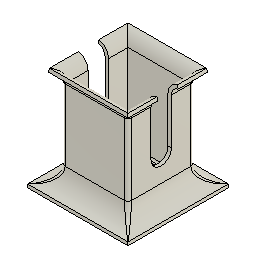
Butter Stick v2 (Autodesk Fusion 360 design; units mm, degrees)
Autodesk Fusion 360 part; units mm, degrees
sketch "Sketch1" plane through (0, 0, 0) normal (0, 0, 1) x (1, 0, 0)
  line L0 (17.5, -17.5) -> (-17.5, -17.5)
  line L1 (-17.5, -17.5) -> (-17.5, 17.5)
  line L2 (-17.5, 17.5) -> (17.5, 17.5)
  line L3 (17.5, 17.5) -> (17.5, -17.5)
  line L4 (17.5, -17.5) -> (-17.5, 17.5) construction
  line L5 (-17.5, -17.5) -> (17.5, 17.5) construction
  dimension "d1" = 35
  dimension "d2" = 35
  constraint perpendicular L0 L1
  constraint parallel L0 L2
  constraint parallel L1 L3
  constraint horizontal L0
  constraint coincident L4 origin
  constraint coincident L5 origin
  measures "d1" distance of L1.end L2.end
  measures "d2" distance of L0.end L1.end
extrude "Extrude1" add sketch "Sketch1" along normal blind 50
shell "Shell1" thickness 2 outward yes removed faces 1 at (5.8333, -5.8333, 50)
sketch "Sketch2" plane through (0, 0, -2) normal (0, 0, -1) x (1, 0, 0)
  line L0 (-19.5, -19.5) -> (19.5, -19.5)
  line L1 (19.5, -19.5) -> (19.5, 19.5)
  line L2 (19.5, 19.5) -> (-19.5, 19.5)
  line L3 (-19.5, 19.5) -> (-19.5, -19.5)
  line L4 (29.5, -29.5) -> (-29.5, -29.5)
  line L5 (-29.5, -29.5) -> (-29.5, 29.5)
  line L6 (-29.5, 29.5) -> (29.5, 29.5)
  line L7 (29.5, 29.5) -> (29.5, -29.5)
  line L8 (29.5, -29.5) -> (-29.5, 29.5) construction
  line L9 (-29.5, -29.5) -> (29.5, 29.5) construction
  dimension "d6" = 10
  constraint perpendicular L4 L5
  constraint parallel L4 L6
  constraint parallel L5 L7
  constraint horizontal L4
  constraint coincident L8 origin
  constraint coincident L9 origin
  measures "d6" distance of L1 L7
extrude "Extrude2" add sketch "Sketch2" along normal blind 2 contours L0 L1 L2 L3 | L4 L5 L6 L7
fillet "Fillet1" radius 10 4 edges at (19.5, 0, -2) (0, 19.5, -2) (-19.5, 0, -2) (0, -19.5, -2)
sketch "Sketch3" plane through (0, 0, 0) normal (1, 0, 0) x (0, 1, 0)
  line L0 (17.5, 0) -> (-17.5, 0)
  line L1 (-17.5, 0) -> (-17.5, 50)
  line L2 (-17.5, 50) -> (17.5, 50)
  line L3 (17.5, 50) -> (17.5, 0)
  line L4 (19.5, 8) -> (19.5, 50)
  line L5 (19.5, 50) -> (19.5, 8)
  arc A0 (23.5, 55) -> (19.5, 50) centre (24.625, 50) ccw
  arc A1 (23.061, 56.9512) -> (17.5, 50) centre (24.625, 50) ccw
  line L6 (24.625, 50) -> (23.061, 56.9512)
  line L7 (19.5, 50) -> (17.5, 50)
  dimension "d16" = 4
  dimension "d17" = 5
  constraint tangent L5 A0
  constraint coincident L4.end L5.start
  constraint tangent L3 A1
  constraint coincident L2.end L3.start
  constraint coincident A0.centre A1.centre
  constraint coincident A0.start L6
  measures "d16" distance of L5 A0.start
  measures "d17" vertical distance of A0.start L4.end
sweep "Sweep1" add profiles "Sketch3" along 4 edges at (-17.5, 0, 50) (0, 17.5, 50) (17.5, 0, 50) (0, -17.5, 50) section 1 contours A0 A1 L6 L7
sketch "Sketch4" plane through (-19.5, 0, 0) normal (-1, 0, 0) x (0, -1, 0)
  line L0 (-19.5, 8) -> (19.5, 8)
  line L1 (19.5, 8) -> (19.5, 50)
  line L2 (19.5, 50) -> (-19.5, 50)
  line L3 (-19.5, 50) -> (-19.5, 8)
  circle A0 centre (-0.0025, 23) radius 6
  line L4 (-6.0025, 23) -> (-6.0025, 56.9512)
  line L5 (5.9975, 23) -> (5.9975, 56.9512)
  line L6 (5.9975, 56.9512) -> (-6.0025, 56.9512)
  line L7 (23.061, 56.9512) -> (-23.061, 56.9512)
  dimension "d18" = 12
  dimension "d19" = 15
  constraint coincident A0 L4.start
  constraint tangent A0 L4
  constraint coincident A0 L5.start
  constraint vertical L5
  constraint tangent A0 L5
  constraint parallel L4 L5
  constraint perpendicular L4 L6
  constraint collinear L6 L7
  measures "d18" diameter of A0
  measures "d19" distance of L0 A0.centre
extrude "Extrude3" cut sketch "Sketch4" along normal through all and the other way through all contours L2 L4 L5 L6 L7 | L2 A0 L4 L5 | A0
sketch "Sketch5" plane through (0, 0, 0) normal (0, 0, 1) x (-1, 0, 0)
  line L0 (-17.5, -17.5) -> (17.5, -17.5)
  line L1 (17.5, -17.5) -> (17.5, 17.5)
  line L2 (17.5, 17.5) -> (-17.5, 17.5)
  line L3 (-17.5, 17.5) -> (-17.5, -17.5)
  line L4 (-2, 2) -> (2, 2)
  line L5 (2, 2) -> (2, -2)
  line L6 (2, -2) -> (-2, -2)
  line L7 (-2, -2) -> (-2, 2)
  line L8 (-2, 2) -> (2, -2) construction
  line L9 (2, 2) -> (-2, -2) construction
  line L10 (-10.5, -14.5) -> (-14.5, -14.5)
  line L11 (-14.5, -14.5) -> (-14.5, -10.5)
  line L12 (-14.5, -10.5) -> (-10.5, -10.5)
  line L13 (-10.5, -10.5) -> (-10.5, -14.5)
  line L14 (-4.25, -14.5) -> (-8.25, -14.5)
  line L15 (-8.25, -14.5) -> (-8.25, -10.5)
  line L16 (-8.25, -10.5) -> (-4.25, -10.5)
  line L17 (-4.25, -10.5) -> (-4.25, -14.5)
  line L18 (2, -14.5) -> (-2, -14.5)
  line L19 (-2, -14.5) -> (-2, -10.5)
  line L20 (-2, -10.5) -> (2, -10.5)
  line L21 (2, -10.5) -> (2, -14.5)
  line L22 (8.25, -14.5) -> (4.25, -14.5)
  line L23 (4.25, -14.5) -> (4.25, -10.5)
  line L24 (4.25, -10.5) -> (8.25, -10.5)
  line L25 (8.25, -10.5) -> (8.25, -14.5)
  line L26 (14.5, -14.5) -> (10.5, -14.5)
  line L27 (10.5, -14.5) -> (10.5, -10.5)
  line L28 (10.5, -10.5) -> (14.5, -10.5)
  line L29 (14.5, -10.5) -> (14.5, -14.5)
  line L30 (-10.5, -8.25) -> (-14.5, -8.25)
  line L31 (-14.5, -8.25) -> (-14.5, -4.25)
  line L32 (-14.5, -4.25) -> (-10.5, -4.25)
  line L33 (-10.5, -4.25) -> (-10.5, -8.25)
  line L34 (-4.25, -8.25) -> (-8.25, -8.25)
  line L35 (-8.25, -8.25) -> (-8.25, -4.25)
  line L36 (-8.25, -4.25) -> (-4.25, -4.25)
  line L37 (-4.25, -4.25) -> (-4.25, -8.25)
  line L38 (2, -8.25) -> (-2, -8.25)
  line L39 (-2, -8.25) -> (-2, -4.25)
  line L40 (-2, -4.25) -> (2, -4.25)
  line L41 (2, -4.25) -> (2, -8.25)
  line L42 (8.25, -8.25) -> (4.25, -8.25)
  line L43 (4.25, -8.25) -> (4.25, -4.25)
  line L44 (4.25, -4.25) -> (8.25, -4.25)
  line L45 (8.25, -4.25) -> (8.25, -8.25)
  line L46 (14.5, -8.25) -> (10.5, -8.25)
  line L47 (10.5, -8.25) -> (10.5, -4.25)
  line L48 (10.5, -4.25) -> (14.5, -4.25)
  line L49 (14.5, -4.25) -> (14.5, -8.25)
  line L50 (-10.5, -2) -> (-14.5, -2)
  line L51 (-14.5, -2) -> (-14.5, 2)
  line L52 (-14.5, 2) -> (-10.5, 2)
  line L53 (-10.5, 2) -> (-10.5, -2)
  line L54 (-4.25, -2) -> (-8.25, -2)
  line L55 (-8.25, -2) -> (-8.25, 2)
  line L56 (-8.25, 2) -> (-4.25, 2)
  line L57 (-4.25, 2) -> (-4.25, -2)
  line L58 (8.25, -2) -> (4.25, -2)
  line L59 (4.25, -2) -> (4.25, 2)
  line L60 (4.25, 2) -> (8.25, 2)
  line L61 (8.25, 2) -> (8.25, -2)
  line L62 (14.5, -2) -> (10.5, -2)
  line L63 (10.5, -2) -> (10.5, 2)
  line L64 (10.5, 2) -> (14.5, 2)
  line L65 (14.5, 2) -> (14.5, -2)
  line L66 (-10.5, 4.25) -> (-14.5, 4.25)
  line L67 (-14.5, 4.25) -> (-14.5, 8.25)
  line L68 (-14.5, 8.25) -> (-10.5, 8.25)
  line L69 (-10.5, 8.25) -> (-10.5, 4.25)
  line L70 (-4.25, 4.25) -> (-8.25, 4.25)
  line L71 (-8.25, 4.25) -> (-8.25, 8.25)
  line L72 (-8.25, 8.25) -> (-4.25, 8.25)
  line L73 (-4.25, 8.25) -> (-4.25, 4.25)
  line L74 (2, 4.25) -> (-2, 4.25)
  line L75 (-2, 4.25) -> (-2, 8.25)
  line L76 (-2, 8.25) -> (2, 8.25)
  line L77 (2, 8.25) -> (2, 4.25)
  line L78 (8.25, 4.25) -> (4.25, 4.25)
  line L79 (4.25, 4.25) -> (4.25, 8.25)
  line L80 (4.25, 8.25) -> (8.25, 8.25)
  line L81 (8.25, 8.25) -> (8.25, 4.25)
  line L82 (14.5, 4.25) -> (10.5, 4.25)
  line L83 (10.5, 4.25) -> (10.5, 8.25)
  line L84 (10.5, 8.25) -> (14.5, 8.25)
  line L85 (14.5, 8.25) -> (14.5, 4.25)
  line L86 (-10.5, 10.5) -> (-14.5, 10.5)
  line L87 (-14.5, 10.5) -> (-14.5, 14.5)
  line L88 (-14.5, 14.5) -> (-10.5, 14.5)
  line L89 (-10.5, 14.5) -> (-10.5, 10.5)
  line L90 (-4.25, 10.5) -> (-8.25, 10.5)
  line L91 (-8.25, 10.5) -> (-8.25, 14.5)
  line L92 (-8.25, 14.5) -> (-4.25, 14.5)
  line L93 (-4.25, 14.5) -> (-4.25, 10.5)
  line L94 (2, 10.5) -> (-2, 10.5)
  line L95 (-2, 10.5) -> (-2, 14.5)
  line L96 (-2, 14.5) -> (2, 14.5)
  line L97 (2, 14.5) -> (2, 10.5)
  line L98 (8.25, 10.5) -> (4.25, 10.5)
  line L99 (4.25, 10.5) -> (4.25, 14.5)
  line L100 (4.25, 14.5) -> (8.25, 14.5)
  line L101 (8.25, 14.5) -> (8.25, 10.5)
  line L102 (14.5, 10.5) -> (10.5, 10.5)
  line L103 (10.5, 10.5) -> (10.5, 14.5)
  line L104 (10.5, 14.5) -> (14.5, 14.5)
  line L105 (14.5, 14.5) -> (14.5, 10.5)
  dimension "d22" = 4
  dimension "d23" = 4
  dimension "d26" = 12.5
  dimension "d27" = 12.5
  constraint perpendicular L4 L5
  constraint parallel L4 L6
  constraint parallel L5 L7
  constraint horizontal L4
  constraint coincident L8 origin
  constraint coincident L9 origin
  measures "d22" distance of L5.end L6.end
  measures "d23" distance of L4.end L5.end
extrude "Extrude4" cut sketch "Sketch5" against normal through all contours L4 L5 L6 L7 | L10 L11 L12 L13 | L14 L15 L16 L17 | L18 L19 L20 L21 | L22 L23 L24 L25 | L26 L27 L28 L29 | L30 L31 L32 L33 | L34 L35 L36 L37 | L38 L39 L40 L41 | L42 L43 L44 L45 | L46 L47 L48 L49 | L50 L51 L52 L53 | L54 L55 L56 L57 | L58 L59 L60 L61 | L62 L63 L64 L65 | L66 L67 L68 L69 | L70 L71 L72 L73 | L74 L75 L76 L77 | L78 L79 L80 L81 | L82 L83 L84 L85 | L86 L87 L88 L89 | L90 L91 L92 L93 | L94 L95 L96 L97 | L98 L99 L100 L101 | L102 L103 L104 L105
fillet "Fillet2" radius 1 1 faces at (-16.5, -0.6667, 0)
fillet "Fillet3" radius 2 12 edges at (20.623, 20.623, 53.2016) (19.5, 19.5, 29) (22.4289, 22.4289, 0.9289) (22.4289, -22.4289, 0.9289) (19.5, -19.5, 29) (20.623, -20.623, 53.2016) (-22.4289, 22.4289, 0.9289) (-19.5, 19.5, 29) (-20.623, 20.623, 53.2016) (-22.4289, -22.4289, 0.9289) (-19.5, -19.5, 29) (-20.623, -20.623, 53.2016)
sketch "Sketch6" plane through (0, 0, 0) normal (0, 0, 1) x (1, 0, 0)
sketch "Sketch8" plane through (0, 0, 0) normal (0, 0, 1) x (1, 0, 0)
  circle A0 centre (0, 0) radius 10
  circle A1 centre (0, 0) radius 11.5
  dimension "d33" = 20
  dimension "d34" = 23
  constraint coincident A0.centre A1.centre
  measures "d33" diameter of A0
  measures "d34" diameter of A1
extrude "Extrude5" add sketch "Sketch8" against normal up to surface (4 mm away)
extrude "Extrude6" cut sketch "Sketch8" against normal through all contours A0
chamfer "Chamfer1" distance 1 angle 45 1 edges at (-9.3233, -3.6162, -4)
